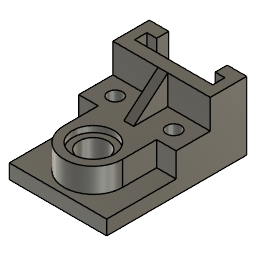
Part1Model (Autodesk Fusion 360 design; units mm, degrees)
part number: 2026-04-19-09-34-39-447
Autodesk Fusion 360 part; units mm, degrees
sketch "Sketch1" plane through (0, 0, 0) normal (0, 0, 1) x (1, 0, 0)
  line L0 (0, 0) -> (80, 0)
  line L1 (80, 0) -> (80, 115)
  line L2 (80, 115) -> (0, 115)
  line L3 (0, 115) -> (0, 0)
  dimension "d1" = 80
  dimension "d2" = 115
  constraint horizontal L0
  constraint vertical L1
  constraint horizontal L2
  constraint vertical L3
  constraint coincident L0.start L3.end
  measures "d1" distance of L0.start L0.end
  measures "d2" distance of L0.start L2.end
sketch "Sketch2" plane through (0, 0, 0) normal (0, 0, 1) x (1, 0, 0)
extrude "Extrude1" add sketch "Sketch1" along normal blind 12
sketch "Sketch3" plane through (0, 0, 12) normal (0, 0, 1) x (-1, 0, 0)
  line L0 (0, -115) -> (0, 0)
  line L1 (0, 0) -> (-80, 0)
  line L2 (-80, 0) -> (-80, -115)
  line L3 (-80, -115) -> (0, -115)
  line L4 (0, -115) -> (-80, -115)
  line L5 (-80, -115) -> (-80, -57)
  line L6 (-80, -57) -> (0, -57)
  line L7 (0, -57) -> (0, -115)
  line L8 (-16, -57) -> (-64, -57)
  line L9 (-64, -57) -> (-64, -29)
  line L10 (-64, -29) -> (-16, -29)
  line L11 (-16, -29) -> (-16, -57)
  circle A0 centre (-40, -29) radius 24
  dimension "d5" = 58
  dimension "d6" = 48
  dimension "d7" = 28
  constraint horizontal L4
  constraint vertical L5
  constraint horizontal L6
  constraint vertical L7
  constraint coincident L0.start L3.end
  constraint horizontal L8
  constraint vertical L9
  constraint horizontal L10
  constraint vertical L11
  constraint coincident L6 L8.start
  constraint midpoint L10 A0.centre
  constraint coincident L9.end A0
  measures "d5" distance of L0.start L6.end
  measures "d6" distance of L8.start L8.end
  measures "d7" distance of L8.start L10.end
extrude "Extrude2" add sketch "Sketch3" along normal blind 20 contours L0 L2 L3 L4 L5 L6 L7 L8 | L6 L8 L9 L11 A0 | L10 A0 | L10 A0
sketch "Sketch4" plane through (0, 0, 32) normal (0, 0, 1) x (-1, 0, 0)
  line L0 (-16, -57) -> (-16, -29)
  arc A0 (-16, -29) -> (-64, -29) centre (-40, -29) ccw
  line L1 (-64, -29) -> (-64, -57)
  line L2 (-64, -57) -> (-80, -57)
  line L3 (-80, -57) -> (-80, -115)
  line L4 (-80, -115) -> (0, -115)
  line L5 (0, -115) -> (0, -57)
  line L6 (0, -57) -> (-16, -57)
  line L7 (0, -115) -> (-80, -115)
  line L8 (-80, -115) -> (-80, -85)
  line L9 (-80, -85) -> (0, -85)
  line L10 (0, -85) -> (0, -115)
  line L11 (-40, -85) -> (-37.1656, -85)
  line L12 (-37.1656, -85) -> (-37.1656, -57)
  line L13 (-37.1656, -57) -> (-40, -57)
  line L14 (-40, -57) -> (-40, -85)
  line L15 (-37.1656, -57) -> (-45.1656, -57)
  line L16 (-45.1656, -57) -> (-45.1656, -85)
  line L17 (-45.1656, -85) -> (-37.1656, -85)
  line L18 (-37.1656, -85) -> (-37.1656, -57)
  dimension "d10" = 28
  dimension "d11" = 8
  constraint horizontal L7
  constraint vertical L8
  constraint horizontal L9
  constraint vertical L10
  constraint coincident L3 L8.end
  constraint coincident L4.end L5.start
  constraint horizontal L11
  constraint vertical L12
  constraint horizontal L13
  constraint vertical L14
  constraint midpoint L9 L11.start
  constraint horizontal L15
  constraint vertical L16
  constraint horizontal L17
  constraint vertical L18
  measures "d10" distance of L11.start L13.end
  measures "d11" distance of L12.end L15.end
extrude "Extrude3" add sketch "Sketch4" along normal blind 24 contours L3 L4 L5 L7 L8 L9 L10 L11 L17 | L9 L11 L12 L13 L14 L15 L17 L18 | L9 L14 L15 L16 L17
sketch "Sketch5" plane through (37.1656, 0, 0) normal (-1, 0, 0) x (0, -1, 0)
  line L0 (-85, 32) -> (-57, 32)
  line L1 (-57, 32) -> (-57, 56)
  line L2 (-57, 56) -> (-85, 56)
  line L3 (-85, 56) -> (-85, 32)
  line L4 (-85, 56) -> (-57, 32)
  line L5 (-85, 56) -> (-57, 56)
  line L6 (-57, 32) -> (-57, 56)
  constraint coincident L2.end L3.start
  constraint coincident L0.end L1.start
  constraint coincident L1.end L2.start
extrude "Extrude4" cut sketch "Sketch5" against normal blind 8 contours L1 L2 L4 L5 L6
sketch "Sketch6" plane through (0, 0, 56) normal (0, 0, 1) x (-1, 0, 0)
  line L0 (-37.1656, -85) -> (-45.1656, -85)
  line L1 (-45.1656, -85) -> (-80, -85)
  line L2 (-80, -85) -> (-80, -115)
  line L3 (-80, -115) -> (0, -115)
  line L4 (0, -115) -> (0, -85)
  line L5 (0, -85) -> (-37.1656, -85)
  line L6 (0, -115) -> (-16, -115)
  line L7 (-16, -115) -> (-16, -105)
  line L8 (-16, -105) -> (-8, -105)
  line L9 (-8, -105) -> (-8, -95)
  line L10 (-80, -115) -> (-64, -115)
  line L11 (-64, -115) -> (-64, -105)
  line L12 (-64, -105) -> (-72, -105)
  line L13 (-72, -105) -> (-72, -95)
  line L14 (-72, -95) -> (-8, -95)
  line L15 (-16, -115) -> (-64, -115)
  dimension "d16" = 16
  dimension "d17" = 10
  dimension "d18" = 10
  dimension "d19" = 16
  dimension "d20" = 8
  constraint coincident L3.end L4.start
  constraint perpendicular L4 L6
  constraint perpendicular L6 L7
  constraint perpendicular L7 L8
  constraint perpendicular L5 L9
  constraint coincident L2.end L3.start
  constraint perpendicular L2 L10
  constraint perpendicular L10 L11
  constraint perpendicular L11 L12
  constraint perpendicular L10 L13
  constraint parallel L12 L14
  measures "d16" distance of L3.end L6.end
  measures "d17" distance of L6.end L7.end
  measures "d18" distance of L8.end L9.end
  measures "d19" distance of L2.end L10.end
  measures "d20" distance of L11.end L12.end
extrude "Extrude5" cut sketch "Sketch6" against normal blind 90 contours L3 L7 L8 L9 L11 L12 L13 L14 L15
sketch "Sketch7" plane through (0, 0, 32) normal (0, 0, 1) x (-1, 0, 0)
  line L0 (-80, -85) -> (-45.1656, -85)
  line L1 (-45.1656, -85) -> (-45.1656, -57)
  line L2 (-45.1656, -57) -> (-37.1656, -57)
  line L3 (-37.1656, -57) -> (-37.1656, -85)
  line L4 (-37.1656, -85) -> (0, -85)
  line L5 (0, -85) -> (0, -57)
  line L6 (0, -57) -> (-16, -57)
  line L7 (-16, -57) -> (-16, -29)
  arc A0 (-16, -29) -> (-64, -29) centre (-40, -29) ccw
  line L8 (-64, -29) -> (-64, -57)
  line L9 (-64, -57) -> (-80, -57)
  line L10 (-80, -57) -> (-80, -85)
  circle A1 centre (-40, -29) radius 17
  dimension "d23" = 34
  constraint concentric A0 A1
  measures "d23" diameter of A1
extrude "Extrude6" cut sketch "Sketch7" against normal blind 5 contours A1
sketch "Sketch8" plane through (0, 0, 27) normal (0, 0, 1) x (-1, 0, 0)
  circle A0 centre (-40, -29) radius 17
  circle A1 centre (-40, -29) radius 12
  dimension "d26" = 24
  constraint concentric A0 A1
  measures "d26" diameter of A1
extrude "Extrude7" cut sketch "Sketch8" against normal blind 49 contours A1
sketch "Sketch9" plane through (0, 0, 32) normal (0, 0, 1) x (-1, 0, 0)
  circle A0 centre (-40, -29) radius 17
  line L0 (-80, -85) -> (-45.1656, -85)
  line L1 (-45.1656, -85) -> (-45.1656, -57)
  line L2 (-45.1656, -57) -> (-37.1656, -57)
  line L3 (-37.1656, -57) -> (-37.1656, -85)
  line L4 (-37.1656, -85) -> (0, -85)
  line L5 (0, -85) -> (0, -57)
  line L6 (0, -57) -> (-16, -57)
  line L7 (-16, -57) -> (-16, -29)
  arc A1 (-16, -29) -> (-64, -29) centre (-40, -29) ccw
  line L8 (-64, -29) -> (-64, -57)
  line L9 (-64, -57) -> (-80, -57)
  line L10 (-80, -57) -> (-80, -85)
  circle A2 centre (-16, -71) radius 6
  circle A3 centre (-64, -71) radius 6
  dimension "d29" = 12
  dimension "d30" = 12
  measures "d29" diameter of A2
  measures "d30" diameter of A3
extrude "Extrude8" cut sketch "Sketch9" against normal blind 46 contours A2 | A3
